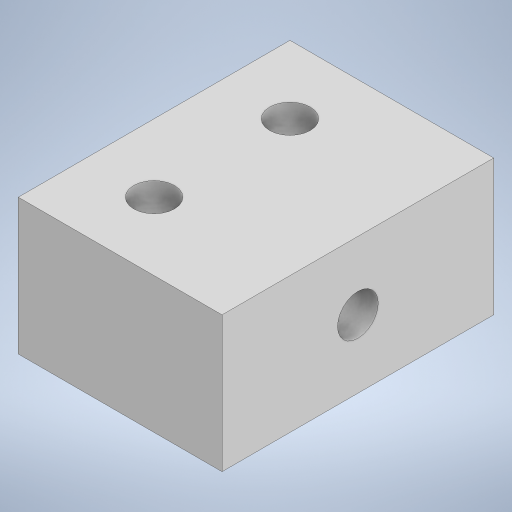
# Autodesk Inventor part: profile1
Saved by Autodesk Inventor 2023 (Build 270158000, 158)
## iProperties
Created: 2024-02-07
Part Number: profile1
Material: Generic
Document SubType Name: Modeling
Designer: victo
Density: 1 g/cm^3
Appearance: Default
Author: victo
Autodesk Inventor part; units mm, degrees
ref_plane "YZ Plane" through (0, 0, 0) normal (1, 0, 0) x (0, 1, 0)
ref_plane "XZ Plane" through (0, 0, 0) normal (0, 1, 0) x (-1, 0, 0)
ref_plane "XY Plane" through (0, 0, 0) normal (0, 0, 1) x (1, 0, 0)
sketch "Sketch1" plane through (0, 0, 0) normal (0, 0, 1) x (1, 0, 0)
  line L0 (0, 0) -> (15, 0)
  line L1 (15, 0) -> (15, 10)
  line L2 (15, 10) -> (0, 10)
  line L3 (0, 10) -> (0, 0)
  line L4 (1, 9) -> (14, 9)
  line L5 (14, 9) -> (14, 1)
  line L6 (14, 1) -> (1, 1)
  line L7 (1, 1) -> (1, 9)
  dimension "d0" = 15
  dimension "d1" = 10
  dimension "d2" = 13
  dimension "d3" = 8
  dimension "d4" = 1
  dimension "d5" = 1
  constraints: 16 end point, 4 parallel, 2 horizontal, 2 perpendicular
  measures "d0" distance of L2.end L1.end
  measures "d1" distance of L1.end L0.end
  measures "d2" distance of L5.end L6.end
  measures "d3" distance of L4.end L5.end
  measures "d4" distance between parallel lines of L3 L7
  measures "d5" distance between parallel lines of L2 L4
extrude "Extrusion1" add sketch "Sketch1" along normal blind 20 contours L3 L2 L1 L0 | L4 L5 L6 L7
sketch "Sketch2" plane through (0, 10, 0) normal (0, 1, 0) x (1, 0, 0)
  line L0 (15, 0) -> (0, 0) projected
  line L1 (0, 0) -> (0, -20) projected
  line L2 (15, -20) -> (0, -20) projected
  line L3 (15, 0) -> (15, -20) projected
  circle A0 centre (5, -5) radius 1.5
  circle A1 centre (5, -15) radius 1.5
  dimension "d8" = 3
  dimension "d9" = 3
  dimension "d10" = 5
  dimension "d11" = 5
  dimension "d12" = 5
  dimension "d13" = 5
  constraints: 2 centre point
  measures "d8" diameter of A0
  measures "d9" diameter of A1
  measures "d10" distance from line of L1 A0.centre
  measures "d11" distance from line of L1 A1.centre
  measures "d12" distance from line of L0 A0.centre
  measures "d13" distance from line of L2 A1.centre
extrude "Extrusion2" cut sketch "Sketch2" against normal up to surface (10 mm away) contours A0 | A1
sketch "Sketch3" plane through (15, 0, 0) normal (1, 0, 0) x (0, 0, -1)
  line L0 (0, 0) -> (0, 10) projected
  line L1 (0, 10) -> (-20, 10) projected
  line L2 (-20, 0) -> (-20, 10) projected
  line L3 (0, 0) -> (-20, 0) projected
  circle A0 centre (-10, 5) radius 1.5
  dimension "d16" = 3
  dimension "d17" = 5
  dimension "d18" = 10
  constraints: 1 centre point
  measures "d16" diameter of A0
  measures "d17" distance from line of L1 A0.centre
  measures "d18" distance from line of L0 A0.centre
extrude "Extrusion3" cut sketch "Sketch3" against normal up to surface (15 mm away) contours A0
body "Solid1"
